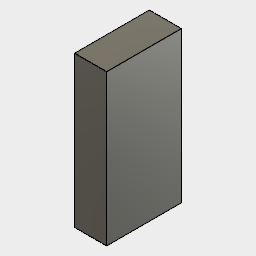
FPROJ_001 (Autodesk Fusion 360 design; units mm, degrees)
Autodesk Fusion 360 part; units mm, degrees
box "长方体基本要素1" add length 46.9727 width 23.2749 height 10 placed x (0, -1, 0) y (0, 0, -1) z (1, 0, 0) at (0, 50, 70)
